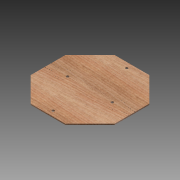
# Autodesk Inventor part: Robot-Lower-Base
Saved by Autodesk Inventor 2012 (Build 160160000, 160)
## iProperties
Created: 2013-07-14
Part Number: Robot-Lower-Base
Material: Wood (Birch)
Document SubType Name: Modeling
Designer: joe_000
Density: 0.55 g/cm^3
Mass: 415.981 g
Surface Area: 2819.96 cm^2
Volume: 756.329 cm^3
BaseSupportThickness: 0.500 in
BaseSupportHeight: 2.661 in
BaseWidth: 16.000 in
BaseSideLength: 6.627 in
Author: joe_000
Autodesk Inventor part; units mm, degrees
ref_plane "YZ Plane" through (0, 0, 0) normal (1, 0, 0) x (0, 1, 0)
ref_plane "XZ Plane" through (0, 0, 0) normal (0, 1, 0) x (-1, 0, 0)
ref_plane "XY Plane" through (0, 0, 0) normal (0, 0, 1) x (1, 0, 0)
sketch "Sketch1" plane through (0, 0, 0) normal (0, 1, 0) x (-1, 0, 0)
  line L0 (-203.2, 84.1682) -> (-84.1682, 203.2)
  line L1 (-84.1682, 203.2) -> (84.1682, 203.2)
  line L2 (84.1682, 203.2) -> (203.2, 84.1682)
  line L3 (203.2, 84.1682) -> (203.2, -84.1682)
  line L4 (203.2, -84.1682) -> (84.1682, -203.2)
  line L5 (84.1682, -203.2) -> (-84.1682, -203.2)
  line L6 (-84.1682, -203.2) -> (-203.2, -84.1682)
  line L7 (-203.2, -84.1682) -> (-203.2, 84.1682)
  point P0 (0, 0)
  point P1 (0, 0)
  dimension "BaseWidth" = 406.4
  dimension "BaseSideLength" = 168.3364
  constraints: 16 end point, 1 coincident, 1 vertical, 17 other
  measures "BaseWidth" distance between parallel lines of L7 L3
  measures "BaseSideLength" distance of L0.end L1.end
extrude "Extrusion1" add sketch "Sketch1" along normal blind 5.5563
sketch "Sketch2" plane through (0, 5.5563, 0) normal (0, 1, 0) x (1, 0, 0)
  line L0 (84.1682, -203.2) -> (-84.1682, -203.2) projected
  line L1 (203.2, 84.1682) -> (203.2, -84.1682) projected
  line L2 (-203.2, -84.1682) -> (-203.2, 84.1682) projected
  line L3 (84.1682, -203.2) -> (-84.1682, -203.2) projected
  line L4 (203.2, 84.1682) -> (203.2, -84.1682) projected
  line L5 (-84.1682, 203.2) -> (84.1682, 203.2) projected
  line L6 (-203.2, -84.1682) -> (-203.2, 84.1682) projected
  line L7 (-203.2, 0) -> (203.2, 0)
  line L8 (0, 203.2) -> (0, -203.2)
  circle A0 centre (-170.025, 15.5) radius 1.75
  circle A1 centre (-180.025, 15.5) radius 1.75
  circle A2 centre (-190.025, 15.5) radius 1.75
  circle A3 centre (-200.025, 15.5) radius 1.75
  circle A4 centre (-170.025, -15.5) radius 1.75
  circle A5 centre (-180.025, -15.5) radius 1.75
  circle A6 centre (-190.025, -15.5) radius 1.75
  circle A7 centre (-200.025, -15.5) radius 1.75
  circle A8 centre (170.025, 15.5) radius 1.75
  circle A9 centre (180.025, 15.5) radius 1.75
  circle A10 centre (190.025, 15.5) radius 1.75
  circle A11 centre (200.025, 15.5) radius 1.75
  circle A12 centre (170.025, -15.5) radius 1.75
  circle A13 centre (180.025, -15.5) radius 1.75
  circle A14 centre (190.025, -15.5) radius 1.75
  circle A15 centre (200.025, -15.5) radius 1.75
  circle A16 centre (0, -177.8) radius 6.1516
  circle A17 centre (0, 177.8) radius 6.1516
  circle A18 centre (-107.95, 0) radius 6.35
  circle A19 centre (107.95, 0) radius 6.35
  dimension "d39" = 3.5
  dimension "d42" = 10
  dimension "d45" = 31
  dimension "d48" = 3.5
  dimension "d51" = 10
  dimension "d54" = 31
  dimension "d57" = 15.5
  dimension "d58" = 3.175
  dimension "d59" = 3.175
  dimension "d60" = 15.5
  dimension "d71" = 12.3031
  dimension "d72" = 12.3031
  dimension "d73" = 25.4
  dimension "d74" = 25.4
  dimension "d75" = 12.7
  dimension "d76" = 95.25
  dimension "d77" = 95.25
  constraints: 20 centre point, 4 end point, 4 midpoint, 4 point on line, 2 horizontal, 2 vertical, 1 equal radius, 28 other
  measures "d39" diameter of A0
  measures "d42" distance of A0.centre A1.centre
  measures "d45" distance of A0.centre A4.centre
  measures "d48" diameter of A8
  measures "d51" distance of A8.centre A9.centre
  measures "d54" distance of A8.centre A12.centre
  measures "d57" distance from line of L7 A0.centre
  measures "d58" distance from line of L2 A3.centre
  measures "d59" distance from line of L1 A11.centre
  measures "d60" distance from line of L7 A11.centre
  measures "d71" diameter of A16
  measures "d72" diameter of A17
  measures "d73" distance from line of L0 A16.centre
  measures "d74" distance from line of L5 A17.centre
  measures "d75" diameter of A18
  measures "d76" distance from line of A18.centre L2
  measures "d77" distance from line of A19.centre L1
extrude "Extrusion2" cut sketch "Sketch2" against normal through all
sketch "Sketch3" plane through (0, 5.5563, 0) normal (0, 1, 0) x (1, 0, 0)
  line L0 (84.1682, -203.2) -> (-84.1682, -203.2) projected
  line L1 (203.2, -84.1682) -> (84.1682, -203.2) projected
  line L2 (203.2, 84.1682) -> (203.2, -84.1682) projected
  line L3 (84.1682, 203.2) -> (203.2, 84.1682) projected
  line L4 (-84.1682, 203.2) -> (84.1682, 203.2) projected
  line L5 (-203.2, 84.1682) -> (-84.1682, 203.2) projected
  line L6 (-203.2, -84.1682) -> (-203.2, 84.1682) projected
  line L7 (-84.1682, -203.2) -> (-203.2, -84.1682) projected
  line L8 (-203.2, 0) -> (203.2, 0)
  line L9 (0, 203.2) -> (0, -203.2)
  point P0 (0, 0)
  constraints: 4 end point, 4 midpoint
sketch "Sketch5" plane through (0, 5.5563, 0) normal (0, 1, 0) x (1, 0, 0)
  circle A0 centre (-107.95, 0) radius 6.35 projected
  line L0 (84.1682, -203.2) -> (-84.1682, -203.2) projected
  line L1 (203.2, 84.1682) -> (203.2, -84.1682) projected
  line L2 (-203.2, -84.1682) -> (-203.2, 84.1682) projected
  circle A1 centre (-137.16, 29.7109) radius 1.5
  circle A2 centre (-124.46, 29.7109) radius 1.5
  circle A3 centre (-137.16, -29.7109) radius 1.5
  circle A4 centre (-124.46, -29.7109) radius 1.5
  point P0 (0, 0)
  dimension "d78" = 66.04
  dimension "d80" = 3
  dimension "d81" = 29.7109
  dimension "d84" = 12.7
  dimension "d87" = 59.4218
  constraints: 4 centre point, 1 horizontal, 1 vertical, 6 other
  measures "d78" distance from line of L2 A1.centre
  measures "d80" diameter of A1
  measures "d81" vertical distance of A0.centre A1.centre
  measures "d84" distance of A1.centre A2.centre
  measures "d87" distance of A1.centre A3.centre
extrude "Extrusion4" cut sketch "Sketch5" against normal through all contours A1 | A2 | A3 | A4
mirror "Mirror1" about plane through (0, 0, 0) normal (1, 0, 0) of "Extrusion4"
equation "\"d71\" = CasterDrillDiameter"
equation "\"d72\" = CasterDrillDiameter"
equation "\"d77\" = d76"
equation "\"d80\" = HoleDiameter"
equation "\"d81\" = 0.5 * ShroudHoldLongSeperation"
equation "\"d84\" = ShroudHoldShortSeperation"
equation "\"d87\" = ShroudHoldLongSeperation"
equation "\"BaseSupportThickness\" = 12.7"
equation "\"CasterDrillDiameter\" = 12.30312"
equation "\"HoleDiameter\" = 3"
equation "\"ShroudHoldLongSeperation\" = 59.421776"
equation "\"ShroudHoldShortSeperation\" = 12.7"
body "Solid1"
